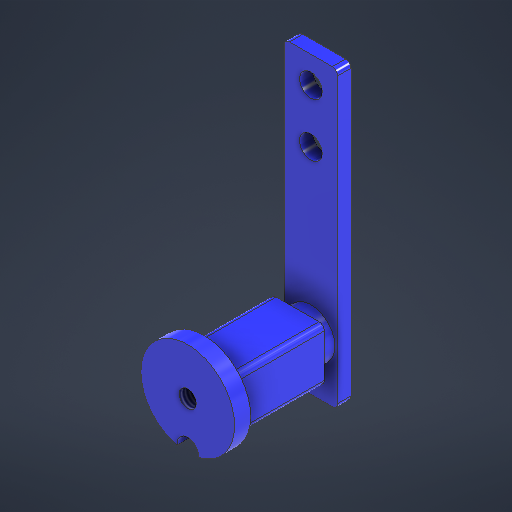
# Autodesk Inventor part: SupportTendeurV2
Saved by Autodesk Inventor 2026.2 (Build 302298010, 298A)
## iProperties
Created: 2026-05-13
Part Number: SupportTendeurV2
Material: Générique
Document SubType Name: Modeling
Designer: romai
Density: 1 g/cm^3
Appearance: Par défaut
Author: romai
Autodesk Inventor part; units mm, degrees
ref_plane "YZ Plane" through (0, 0, 0) normal (1, 0, 0) x (0, 1, 0)
ref_plane "XZ Plane" through (0, 0, 0) normal (0, 1, 0) x (-1, 0, 0)
ref_plane "XY Plane" through (0, 0, 0) normal (0, 0, 1) x (1, 0, 0)
sketch "Esquisse1" plane through (0, 0, 0) normal (0, 0, 1) x (1, 0, 0)
  line L0 (-8, -55) -> (8, -55)
  line L1 (10, -53) -> (10, 53)
  line L2 (8, 55) -> (-8, 55)
  line L3 (-10, 53) -> (-10, -53)
  line L4 (-10, -55) -> (10, 55) construction
  line L5 (10, -55) -> (-10, 55) construction
  arc A0 (-8, 55) -> (-10, 53) centre (-8, 53) ccw
  arc A1 (-10, -53) -> (-8, -55) centre (-8, -53) ccw
  arc A2 (8, -55) -> (10, -53) centre (8, -53) ccw
  arc A3 (10, 53) -> (8, 55) centre (8, 53) ccw
  circle A4 centre (0, 45) radius 4.25
  circle A5 centre (0, 25) radius 4.25
  point P0 (0, 0)
  dimension "d0" = 20
  dimension "d1" = 110
  dimension "d2" = 2
  dimension "d3" = 8.5
  dimension "d4" = 8.5
  dimension "d5" = 80
  dimension "d6" = 20
  constraints: 12 end point, 8 point on circle, 8 point on line, 8 tangent, 6 centre point, 3 equal radius, 2 midpoint, 2 parallel, 1 horizontal, 1 perpendicular
  measures "d0" distance of L5.end L4.end
  measures "d1" distance of L4.end L5.start
  measures "d2" radius of A0
  measures "d3" diameter of A4
  measures "d4" diameter of A5
  measures "d5" distance from line of L0 A5.centre
  measures "d6" distance of A5.centre A4.centre
extrude "Extrusion1" add sketch "Esquisse1" against normal blind 5
sketch "Esquisse2" plane through (0, 0, 0) normal (0, 0, 1) x (1, 0, 0)
  circle A0 centre (0, -35) radius 9
  line L0 (-8, -55) -> (8, -55) projected
  point P0 (0, 0)
  dimension "d9" = 18
  dimension "d10" = 20
  constraints: 1 centre point
  measures "d9" diameter of A0
  measures "d10" distance from line of L0 A0.centre
extrude "Extrusion2" add sketch "Esquisse2" along normal blind 5
sketch "Esquisse3" plane through (0, -35, 5) normal (0, 0, 1) x (1, 0, 0)
  line L0 (-8, 10) -> (8, 10)
  line L1 (10, 8) -> (10, -8)
  line L2 (8, -10) -> (-8, -10)
  line L3 (-10, -8) -> (-10, 8)
  line L4 (-10, 10) -> (10, -10) construction
  line L5 (10, 10) -> (-10, -10) construction
  arc A0 (-8, 10) -> (-10, 8) centre (-8, 8) ccw
  arc A1 (-10, -8) -> (-8, -10) centre (-8, -8) ccw
  arc A2 (8, -10) -> (10, -8) centre (8, -8) ccw
  arc A3 (10, 8) -> (8, 10) centre (8, 8) ccw
  point P0 (0, 35)
  point P1 (0, 0)
  dimension "d13" = 20
  dimension "d14" = 20
  dimension "d17" = 2
  constraints: 12 end point, 8 point on circle, 8 point on line, 8 tangent, 4 centre point, 3 equal radius, 2 midpoint, 2 parallel, 1 horizontal, 1 perpendicular
  measures "d13" distance of L4.end L5.end
  measures "d14" distance of L5.start L4.end
  measures "d17" radius of A0
extrude "Extrusion3" add sketch "Esquisse3" along normal blind 35
sketch "Esquisse4" plane through (0, -35, 40) normal (0, 0, 1) x (1, 0, 0)
  arc A0 (3.9626, -15.4418) -> (-3.9626, -15.4418) centre (0, 1.6036) ccw
  arc A1 (3.9626, -15.4418) -> (-3.9626, -15.4418) centre (0, -14.8964) ccw
  point P0 (0, 35)
  dimension "d18" = 35
  dimension "d19" = 8
  dimension "d20" = 16.5
  constraints: 4 point on circle, 2 centre point
  measures "d18" diameter of A0
  measures "d19" diameter of A1
  measures "d20" distance of A1.centre A0.centre
extrude "Extrusion4" add sketch "Esquisse4" along normal blind 6
sketch "Esquisse5" plane through (0, -35, 46) normal (0, 0, 1) x (1, 0, 0)
  arc A0 (3.9626, -15.4418) -> (-3.9626, -15.4418) centre (0, 1.6036) ccw projected
  point P0 (0, 35)
  constraints: 1 coincident
hole "Perçage1" at (0, -33.3964, 46) direction (0, 0, -1) diameter 6.4008 depth 10 counterbore diameter 12.6 counterbore depth 0 thread size "5/16-18 UNC" class "2B" standard "ANSI Unified Screw Threads"
